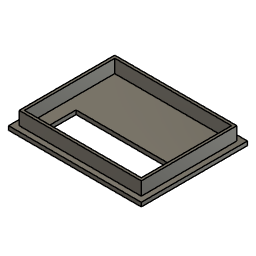
Lid cover v4 (Autodesk Fusion 360 design; units mm, degrees)
Autodesk Fusion 360 part; units mm, degrees
note: some values were not read from the file. Set by a fixed rule: which sketch regions a step uses.
sketch "Sketch1" plane through (0, 0, 0) normal (0, 1, 0) x (1, 0, 0)
  line L0 (50, -40) -> (-50, -40)
  line L1 (-50, -40) -> (-50, 40)
  line L2 (-50, 40) -> (50, 40)
  line L3 (50, 40) -> (50, -40)
  line L4 (50, -40) -> (-50, 40) construction
  line L5 (-50, -40) -> (50, 40) construction
  dimension "d1" = 100
  dimension "d2" = 80
  constraint horizontal L0
  constraint perpendicular L0 L1
  constraint parallel L0 L2
  constraint parallel L1 L3
  constraint coincident L4 origin
  constraint coincident L5 origin
  measures "d1" distance of L1.end L2.end
  measures "d2" distance of L0.end L1.end
extrude "Extrude1" add sketch "Sketch1" along normal blind 3
sketch "Sketch5" plane through (0, 3, 0) normal (0, 1, 0) x (-1, 0, 0)
  line L0 (-50, -40) -> (50, -40)
  line L1 (50, -40) -> (50, 40)
  line L2 (50, 40) -> (-50, 40)
  line L3 (-50, 40) -> (-50, -40)
  line L4 (46, -36) -> (-46, -36)
  line L5 (-46, -36) -> (-46, 36)
  line L6 (-46, 36) -> (46, 36)
  line L7 (46, 36) -> (46, -36)
  line L8 (44, -34) -> (-44, -34)
  line L9 (-44, -34) -> (-44, 34)
  line L10 (-44, 34) -> (44, 34)
  line L11 (44, 34) -> (44, -34)
  dimension "d25" = 72
  dimension "d26" = 92
  dimension "d27" = 4
  dimension "d28" = 4
  dimension "d29" = 4
  dimension "d32" = 4
  dimension "d33" = 2
  dimension "d34" = 2
  dimension "d35" = 88
  dimension "d36" = 68
  constraint horizontal L4
  constraint vertical L5
  constraint horizontal L6
  constraint vertical L7
  constraint horizontal L8
  constraint vertical L9
  constraint horizontal L10
  constraint vertical L11
  measures "d25" distance of L4 L6
  measures "d26" distance of L5 L7
  measures "d27" distance of L3 L5
  measures "d28" distance of L1 L7
  measures "d29" distance of L2 L6
  measures "d32" distance of L0 L4
  measures "d33" distance of L7 L11
  measures "d34" distance of L4 L8
  measures "d35" distance of L9.end L10.end
  measures "d36" distance of L8.end L9.end
extrude "Extrude6" add sketch "Sketch5" along normal blind 10 contours L4 L5 L6 L7
sketch "Sketch6" plane through (0, 0, 0) normal (0, -1, 0) x (1, 0, 0)
  line L0 (-50, -40) -> (50, -40)
  line L1 (50, -40) -> (50, 40)
  line L2 (50, 40) -> (-50, 40)
  line L3 (-50, 40) -> (-50, -40)
  arc A0 (-32, 22.9645) -> (-32.25, 22.7145) centre (-32, 22.7145) ccw
  arc A1 (32.25, 22.7145) -> (32, 22.9645) centre (32, 22.7145) ccw
  arc A2 (-32.25, 8.7145) -> (-32, 8.4645) centre (-32, 8.7145) ccw
  arc A3 (32, 8.4645) -> (32.25, 8.7145) centre (32, 8.7145) ccw
  arc A4 (35.35, 27.1145) -> (34.85, 27.6145) centre (34.85, 27.1145) ccw
  arc A5 (34.85, 3.8145) -> (35.35, 4.3145) centre (34.85, 4.3145) ccw
  arc A6 (-34.85, 27.6145) -> (-35.35, 27.1145) centre (-34.85, 27.1145) ccw
  arc A7 (-35.35, 4.3145) -> (-34.85, 3.8145) centre (-34.85, 4.3145) ccw
  line L4 (35.35, 27.1145) -> (35.35, 4.3145)
  line L5 (34.85, 3.8145) -> (-34.85, 3.8145)
  line L6 (-35.35, 4.3145) -> (-35.35, 27.1145)
  line L7 (-34.85, 27.6145) -> (34.85, 27.6145)
  line L8 (-34.85, 27.1145) -> (35.35, 27.1145)
  line L9 (35.35, 27.1145) -> (35.35, 4.3145)
  line L10 (35.35, 4.3145) -> (-34.85, 4.3145)
  line L11 (-34.85, 4.3145) -> (-34.85, 27.1145)
  constraint horizontal L8
  constraint vertical L9
  constraint horizontal L10
  constraint vertical L11
  constraint coincident A5.end L4.end
  constraint coincident A6.centre L8.start
extrude "Extrude7" cut sketch "Sketch6" against normal blind 10 contours L4 L8 L9 L10 L11
extrude "Extrude2" [suppressed]
sketch "Sketch3" plane through (0, 0, 0) normal (0, -1, 0) x (1, 0, 0)
  line L0 (-50, -40) -> (50, -40)
  line L1 (50, -40) -> (50, 40)
  line L2 (50, 40) -> (-50, 40)
  line L3 (-50, 40) -> (-50, -40)
  line L4 (-32.25, 29.2699) -> (32.25, 29.2699)
  line L5 (32.25, 29.2699) -> (32.25, 13.2699)
  line L6 (32.25, 13.2699) -> (-32.25, 13.2699)
  line L7 (-32.25, 13.2699) -> (-32.25, 29.2699)
  dimension "d11" = 64.5
  dimension "d12" = 16
  dimension "d13" = 17.75
  dimension "d14" = 17.75
  constraint horizontal L4
  constraint vertical L5
  constraint horizontal L6
  constraint vertical L7
  measures "d11" distance of L4.start L4.end
  measures "d12" distance of L4.end L5.end
  measures "d13" distance of L3 L7
  measures "d14" distance of L1 L5
extrude "Extrude3" [suppressed]
sketch "Sketch4" plane through (0, 0, 0) normal (0, -1, 0) x (1, 0, 0)
  line L0 (32.25, 29.2699) -> (32.25, 13.2699)
  line L1 (32.25, 13.2699) -> (-32.25, 13.2699)
  line L2 (-32.25, 13.2699) -> (-32.25, 29.2699)
  line L3 (-32.25, 29.2699) -> (32.25, 29.2699)
  line L4 (-50, -40) -> (50, -40)
  line L5 (50, -40) -> (50, 40)
  line L6 (50, 40) -> (-50, 40)
  line L7 (-50, 40) -> (-50, -40)
  line L8 (-29.2629, -30.2654) -> (30.7371, -30.2654) construction
  line L9 (30.7371, -30.2654) -> (30.7371, -10.2654) construction
  line L10 (30.7371, -10.2654) -> (-29.2629, -10.2654) construction
  line L11 (-29.2629, -10.2654) -> (-29.2629, -30.2654) construction
  dimension "d17" = 7
extrude "Extrude4" [suppressed]
extrude "Extrude5" [suppressed]
